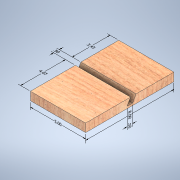
# Autodesk Inventor part: kindleStand
Saved by Autodesk Inventor 2020.2 (Build 242310000, 310)
## iProperties
Created: 2020-01-24
Part Number: kindleStand
Material: Wood (Birch)
Document SubType Name: Modeling
Designer: steele
Density: 0.55 g/cm^3
Appearance: Birch - Natural Polished
Author: steele
Autodesk Inventor part; units mm, degrees
ref_plane "YZ Plane" through (0, 0, 0) normal (1, 0, 0) x (0, 1, 0)
ref_plane "XZ Plane" through (0, 0, 0) normal (0, 1, 0) x (-1, 0, 0)
ref_plane "XY Plane" through (0, 0, 0) normal (0, 0, 1) x (1, 0, 0)
sketch "Sketch2" plane through (0, 0, 0) normal (0, 1, 0) x (-1, 0, 0)
  line L0 (63.5, 101.6) -> (-63.5, 101.6)
  line L1 (-63.5, 101.6) -> (-63.5, -101.6)
  line L2 (-63.5, -101.6) -> (63.5, -101.6)
  line L3 (63.5, -101.6) -> (63.5, 101.6)
  line L4 (63.5, 101.6) -> (-63.5, -101.6) construction
  line L5 (-63.5, 101.6) -> (63.5, -101.6) construction
  point P0 (0, 0)
  dimension "d0" = 127
  dimension "d1" = 203.2
  constraints: 12 end point, 2 midpoint, 2 parallel, 1 horizontal, 1 perpendicular
  measures "d0" distance of L0.start L0.end
  measures "d1" distance of L1.end L0.end
extrude "Extrusion1" add sketch "Sketch2" along normal blind 19.05
sketch "Sketch3" plane through (63.5, 0, 101.6) normal (1, 0, 0) x (0, 0, -1)
  line L0 (101.6, 0) -> (101.6, 19.05) construction
  line L1 (203.2, 19.05) -> (0, 19.05) construction
  line L2 (101.6, 4.8782) -> (107.95, 4.8782)
  line L3 (107.95, 4.8782) -> (116.1321, 19.05)
  line L4 (101.6, 4.8782) -> (95.25, 4.8782)
  line L5 (95.25, 4.8782) -> (103.4321, 19.05)
  line L6 (103.4321, 19.05) -> (116.1321, 19.05)
  dimension "d4" = 6.35
  dimension "d5" = 120
  dimension "d6" = 6.35
  constraints: 12 end point, 3 horizontal, 3 point on line, 1 midpoint, 1 parallel
  measures "d4" distance of L2.start L2.end
  measures "d5" angle of L3 L2
  measures "d6" distance of L2.start L4.end
extrude "Extrusion2" cut sketch "Sketch3" against normal through all
body "Solid1"
